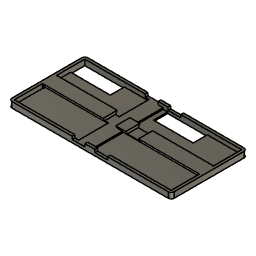
Top Side Cover 2x1 v2 (Autodesk Fusion 360 design; units mm, degrees)
Autodesk Fusion 360 part; units mm, degrees
sketch "Schizzo1" plane through (0, 0, 0) normal (0, 0, 1) x (1, 0, 0)
  line L0 (4.4965, 58.7959) -> (119.1965, 58.7959) construction
  line L1 (119.1965, 58.7959) -> (119.1965, 5.0959) construction
  line L2 (119.1965, 5.0959) -> (4.4965, 5.0959) construction
  line L3 (4.4965, 5.0959) -> (4.4965, 58.7959) construction
  line L4 (4.4965, 31.9459) -> (119.1965, 31.9459) construction
  line L5 (61.8465, 58.7959) -> (61.8465, 5.0959) construction
  line L6 (119.0965, 5.1959) -> (4.5965, 5.1959)
  line L7 (4.5965, 5.1959) -> (4.5965, 58.6959)
  line L8 (4.5965, 58.6959) -> (119.0965, 58.6959)
  line L9 (119.0965, 58.6959) -> (119.0965, 5.1959)
  line L10 (117.1965, 7.0959) -> (6.4965, 7.0959)
  line L11 (6.4965, 7.0959) -> (6.4965, 56.7959)
  line L12 (6.4965, 56.7959) -> (117.1965, 56.7959)
  line L13 (117.1965, 56.7959) -> (117.1965, 7.0959)
  line L14 (6.4965, 56.7959) -> (34.4965, 56.7959)
  line L15 (34.4965, 56.7959) -> (34.4965, 46.7959)
  line L16 (34.4965, 46.7959) -> (6.4965, 46.7959)
  line L17 (6.4965, 46.7959) -> (6.4965, 56.7959)
  line L18 (92.9965, 56.7959) -> (92.9965, 46.7959)
  line L19 (92.9965, 46.7959) -> (64.9965, 46.7959)
  line L20 (64.9965, 46.7959) -> (64.9965, 56.7959)
  line L21 (64.9965, 56.7959) -> (92.9965, 56.7959)
  line L22 (4.4965, 36.9459) -> (119.0965, 36.9459)
  line L23 (4.4965, 26.9459) -> (119.0965, 26.9459)
  line L24 (51.8465, 58.7959) -> (51.8465, 5.0959)
  line L25 (61.8465, 58.7959) -> (61.8465, 5.0959)
  dimension "d1" = 114.7
  dimension "d2" = 53.7
  dimension "d3" = 0.1
  dimension "d6" = 2
  dimension "d7" = 28
  dimension "d8" = 10
  dimension "d11" = 58.5
  dimension "d12" = 0
  dimension "d15" = 10
  dimension "d23" = 10
  constraint horizontal L0
  constraint vertical L1
  constraint horizontal L2
  constraint vertical L3
  constraint midpoint L3 L4.start
  constraint midpoint L1 L4.end
  constraint midpoint L0 L5.start
  constraint midpoint L2 L5.end
  constraint horizontal L14
  constraint vertical L15
  constraint horizontal L16
  constraint vertical L17
  constraint coincident L3 L22.start
  constraint coincident L9 L22.end
  constraint perpendicular L9 L22
  constraint symmetric L4 L22.start L23.start
  constraint symmetric L4 L22.end L23.end
  constraint coincident L0 L24.start
  constraint coincident L2 L24.end
  constraint perpendicular L2 L24
  measures "d1" distance of L1 L3
  measures "d2" distance of L0 L2
  measures "d7" distance of L11.end L14.end
  measures "d8" distance of L11.end L16.end
  measures "d15" distance of L22 L23
  measures "d23" distance of L5 L24
extrude "Estrusione1" add sketch "Schizzo1" along normal blind 1 contours L10 L13 L23 L25 | L10 L23 L24 L25 | L13 L22 L23 L25 | L10 L11 L23 L24 | L22 L23 L24 L25 | L12 L13 L18 L19 L20 L22 L25 | L11 L22 L23 L24 | L12 L22 L24 L25 | L11 L12 L15 L16 L22 L24
extrude "Estrusione2" add sketch "Schizzo1" along normal blind 4 contours L6 L9 L10 L13 L23 L25 | L6 L10 L24 L25 | L9 L13 L22 L23 | L6 L7 L10 L11 L23 L24 | L8 L9 L12 L13 L21 L22 L25 | L13 L22 L23 L25 | L22 L23 L24 L25 | L7 L11 L22 L23 | L11 L22 L23 L24 | L8 L12 L24 L25 | L7 L8 L11 L12 L14 L17 L22 L24
fillet "Raccordo1" radius 2 4 edges at (4.5965, 5.1959, 2) (119.0965, 5.1959, 2) (119.0965, 58.6959, 2) (4.5965, 58.6959, 2)
ref_plane "Piano di lavoro1" through (61.8465, 31.9459, 0) normal (-1, 0, 0) x (0, -1, 0)
sketch "Schizzo3" plane through (61.8465, 0, 0) normal (-1, 0, 0) x (0, -1, 0)
  line L0 (-26.9459, 4) -> (-36.9459, 4) construction
  line L1 (-36.9459, 4) -> (-36.9459, 0) construction
  line L2 (-36.9459, 0) -> (-26.9459, 0) construction
  line L3 (-26.9459, 0) -> (-26.9459, 4) construction
  line L4 (-56.6959, 4) -> (-7.1959, 4) construction
  line L5 (-58.7959, 0) -> (-5.0959, 0) construction
  line L6 (-26.9459, 1) -> (-26.9459, 4) construction
  line L7 (-36.9459, 1) -> (-36.9459, 4) construction
  line L8 (-31.9459, 4) -> (-31.9459, 0) construction
  line L9 (-26.9459, 1) -> (-36.9459, 1) construction
  line L10 (-26.9459, 1) -> (-26.9459, 4)
  line L11 (-26.9459, 4) -> (-28.678, 1)
  line L12 (-28.678, 1) -> (-26.9459, 1)
  line L13 (-36.9459, 1) -> (-36.9459, 4)
  line L14 (-36.9459, 4) -> (-35.2139, 1)
  line L15 (-35.2139, 1) -> (-36.9459, 1)
  dimension "d20" = 30
  constraint horizontal L0
  constraint vertical L1
  constraint horizontal L2
  constraint vertical L3
  constraint collinear L0 L4
  constraint collinear L2 L5
  constraint collinear L3 L6
  constraint collinear L1 L7
  constraint midpoint L4 L8.start
  constraint midpoint L5 L8.end
  constraint coincident L6.start L9.start
  constraint coincident L7.start L9.end
  constraint coincident L0.start L3.end
  constraint coincident L9 L11.end
  constraint symmetric L8 L6.start L7.start
  constraint symmetric L8 L0.start L0.end
  constraint symmetric L8 L11.end L14.end
  measures "d20" angle of L10 L11
extrude "Estrusione4" cut sketch "Schizzo3" along normal mid plane 110
extrude "Estrusione5" add sketch "Schizzo1" along normal blind 2 contours L6 L10 L24 L25 | L10 L23 L24 L25 | L22 L23 L24 L25 | L12 L22 L24 L25 | L8 L12 L24 L25
sketch "Schizzo4" plane through (0, 0, 4) normal (0, 0, 1) x (-1, 0, 0)
  arc A0 (-6.5965, -58.6959) -> (-4.5965, -56.6959) centre (-6.5965, -56.6959) ccw
  line L0 (-4.5965, -56.6959) -> (-4.5965, -7.1959)
  arc A1 (-4.5965, -7.1959) -> (-6.5965, -5.1959) centre (-6.5965, -7.1959) ccw
  line L1 (-6.5965, -5.1959) -> (-117.0965, -5.1959)
  arc A2 (-117.0965, -5.1959) -> (-119.0965, -7.1959) centre (-117.0965, -7.1959) ccw
  line L2 (-119.0965, -7.1959) -> (-119.0965, -56.6959)
  arc A3 (-119.0965, -56.6959) -> (-117.0965, -58.6959) centre (-117.0965, -56.6959) ccw
  line L3 (-117.0965, -58.6959) -> (-6.5965, -58.6959)
  line L4 (-117.1965, -36.9459) -> (-116.8465, -36.9459)
  line L5 (-116.8465, -36.9459) -> (-6.8465, -36.9459)
  line L6 (-6.8465, -36.9459) -> (-6.4965, -36.9459)
  line L7 (-6.4965, -36.9459) -> (-6.4965, -56.7959)
  line L8 (-6.4965, -56.7959) -> (-117.1965, -56.7959)
  line L9 (-117.1965, -56.7959) -> (-117.1965, -36.9459)
  line L10 (-117.1965, -7.0959) -> (-6.4965, -7.0959)
  line L11 (-6.4965, -7.0959) -> (-6.4965, -26.9459)
  line L12 (-6.4965, -26.9459) -> (-6.8465, -26.9459)
  line L13 (-6.8465, -26.9459) -> (-116.8465, -26.9459)
  line L14 (-116.8465, -26.9459) -> (-117.1965, -26.9459)
  line L15 (-117.1965, -26.9459) -> (-117.1965, -7.0959)
  line L16 (-4.5965, -58.6959) -> (-119.0965, -58.6959) construction
  line L17 (-119.0965, -58.6959) -> (-119.0965, -5.1959) construction
  line L18 (-119.0965, -5.1959) -> (-4.5965, -5.1959) construction
  line L19 (-4.5965, -5.1959) -> (-4.5965, -58.6959) construction
  line L20 (-49.1965, -58.6959) -> (-58.1965, -58.6959)
  line L21 (-58.1965, -58.6959) -> (-58.1965, -5.1959)
  line L22 (-58.1965, -5.1959) -> (-49.1965, -5.1959)
  line L23 (-49.1965, -5.1959) -> (-49.1965, -58.6959)
  line L24 (-65.1965, -58.6959) -> (-74.1965, -58.6959)
  line L25 (-74.1965, -58.6959) -> (-74.1965, -5.1959)
  line L26 (-74.1965, -5.1959) -> (-65.1965, -5.1959)
  line L27 (-65.1965, -5.1959) -> (-65.1965, -58.6959)
  line L28 (-53.6965, -58.6959) -> (-53.6965, -5.1959) construction
  line L29 (-69.6965, -58.6959) -> (-69.6965, -5.1959) construction
  line L30 (-2.6965, -58.6959) -> (-2.6965, -5.1959) construction
  dimension "d28" = 9
  dimension "d29" = 9
  dimension "d33" = 1.9
  dimension "d34" = 51
  dimension "d35" = 67
  constraint horizontal L16
  constraint vertical L17
  constraint horizontal L18
  constraint vertical L19
  constraint collinear L3 L16
  constraint collinear L0 L19
  constraint collinear L1 L18
  constraint collinear L2 L17
  constraint horizontal L20
  constraint vertical L21
  constraint horizontal L22
  constraint vertical L23
  constraint coincident L18 L21.end
  constraint coincident L16 L20.start
  constraint horizontal L24
  constraint vertical L25
  constraint horizontal L26
  constraint vertical L27
  constraint coincident L18 L25.end
  constraint coincident L3 L24.start
  constraint midpoint L20 L28.start
  constraint midpoint L22 L28.end
  constraint midpoint L24 L29.start
  constraint midpoint L26 L29.end
  constraint perpendicular L8 L30
  constraint coincident L16 L30.start
  constraint coincident L18 L30.end
  measures "d28" distance of L21 L23
  measures "d29" distance of L25 L27
  measures "d33" distance of L19 L30
  measures "d34" distance of L28 L30
  measures "d35" distance of L29 L30
extrude "Estrusione6" cut sketch "Schizzo4" against normal blind 2 contours L3 L8 L20 L21 L23 | L5 L8 L21 L23 | L3 L8 L24 L25 L27 | L5 L13 L21 L23 | L1 L10 L21 L22 L23 | L5 L8 L25 L27 | L10 L13 L21 L23 | L5 L13 L25 L27 | L1 L10 L25 L26 L27 | L10 L13 L25 L27
